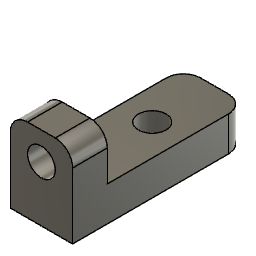
desk_krep (Autodesk Fusion 360 design; units mm, degrees)
Autodesk Fusion 360 part; units mm, degrees
sketch "Sketch1" plane through (0, 0, 0) normal (1, 0, 0) x (0, 0, -1)
  line L0 (0, 0) -> (-25, 0)
  line L1 (-25, 0) -> (-25, 11)
  line L2 (-25, 11) -> (-20, 11)
  line L3 (0, 5) -> (0, 0)
  line L4 (0, 0) -> (0, 5)
  line L5 (-20, 5) -> (-20, 11)
  line L6 (-20, 5) -> (0, 5)
  point P0 (0, 5)
  point P1 (-20, 11)
  point P2 (-20, 5)
  point P3 (-25, 11)
  point P4 (-25, 0)
  constraint horizontal L0
  constraint vertical L1
  constraint horizontal L2
  constraint vertical L3
  constraint coincident L0.start L3.end
  constraint perpendicular L0 L4
  constraint perpendicular L2 L5
  constraint perpendicular L4 L6
  constraint coincident P0 L3.start
  constraint coincident P1 L2.end
  constraint coincident P2 L5.start
  constraint coincident L1.end L2.start
  constraint coincident P4 L0.end
extrude "Extrude1" add sketch "Sketch1" along normal blind 9
sketch "Sketch2" plane through (0, 0, 20) normal (0, 0, -1) x (-1, 0, 0)
  line L0 (0, 5) -> (0, 11)
  line L1 (0, 11) -> (-9, 11)
  line L2 (-9, 11) -> (-9, 5)
  line L3 (-9, 5) -> (0, 5)
  circle A0 centre (-4.5, 8) radius 2
  dimension "d9" = 4
  dimension "d11" = 4.5
  measures "d9" diameter of A0
  measures "d11" horizontal distance of L1.end A0.centre
sketch "Sketch3" plane through (0, 5, 0) normal (0, 1, 0) x (-1, 0, 0)
  line L0 (0, 0) -> (0, 20)
  line L1 (0, 20) -> (-9, 20)
  line L2 (-9, 20) -> (-9, 0)
  line L3 (-9, 0) -> (0, 0)
  circle A0 centre (-4.5, 9) radius 2
  dimension "d12" = 4
  dimension "d14" = 4.5
  measures "d12" diameter of A0
  measures "d14" horizontal distance of L0.start A0.centre
extrude "Extrude2" cut sketch "Sketch3" against normal blind 13 contours A0
extrude "Extrude3" cut sketch "Sketch2" against normal blind 11 contours A0
fillet "Fillet1" radius 2.5 1 edges at (0, 2.5, 0)
fillet "Fillet2" radius 2.5 1 edges at (9, 2.5, 0)
extrude "Extrude4" add 1 faces at (6, 11, 23.3333) along direction (0, 1, 0) blind 1
fillet "Fillet3" radius 2.5 1 edges at (0, 12, 22.5)
fillet "Fillet4" radius 2.5 1 edges at (9, 12, 22.5)
